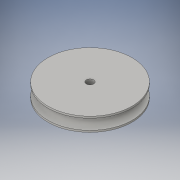
# Autodesk Inventor part: wheel
Saved by Autodesk Inventor 2016 (Build 200138000, 138)
## iProperties
Created: 2019-02-22
Part Number: wheel
Material: Generic
Document SubType Name: Modeling
Designer: davism846
Density: 1 g/cm^3
Appearance: Default
Author: davism846
Autodesk Inventor part; units mm, degrees
ref_plane "YZ Plane" through (0, 0, 0) normal (1, 0, 0) x (0, 1, 0)
ref_plane "XZ Plane" through (0, 0, 0) normal (0, 1, 0) x (-1, 0, 0)
ref_plane "XY Plane" through (0, 0, 0) normal (0, 0, 1) x (1, 0, 0)
sketch "Sketch1" plane through (0, 0, 0) normal (0, 0, 1) x (1, 0, 0)
  line L0 (0, 0) -> (-19.05, 0)
  line L1 (-19.05, 6.35) -> (0, 6.35)
  line L2 (0, 6.35) -> (0, 0)
  line L3 (-19.05, 0) -> (-19.05, 0.7937)
  line L4 (-19.05, 5.5563) -> (-19.05, 6.35)
  line L5 (-19.05, 5.5563) -> (-17.1348, 5.5563)
  arc A0 (-19.05, 0.7937) -> (-19.05, 5.5563) centre (-19.05, 3.175) ccw
  dimension "d0" = 19.05
  dimension "d1" = 6.35
  dimension "d4" = 2.3813
  constraints: 12 end point, 3 parallel, 2 horizontal, 2 perpendicular, 2 point on circle, 1 centre point, 1 tangent
  measures "d0" distance of L1.start L1.end
  measures "d1" distance of L0.end L1.start
  measures "d4" radius of A0
revolve "Revolution1" add sketch "Sketch1" angle 360 about axis through (0, 6.35, 0) along (0, -1, 0)
sketch "Sketch2" plane through (0, 6.35, 0) normal (0, 1, 0) x (1, 0, 0)
  point P0 (0, 0)
  point P1 (0, 0)
  constraints: 1 coincident
hole "Hole1" at (0, 6.35, 0) direction (0, -1, 0) diameter 3.302 end through all
body "Solid1"
